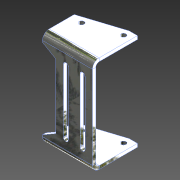
# Autodesk Inventor part: trackball_l
Saved by Autodesk Inventor 2018 (Build 220112000, 112)
## iProperties
Created: 2018-07-04
Part Number: trackball_l
Material: アルミニウム 6061
Document SubType Name: Sheet Metal
Designer: NaMACHAN
Mass: 10.2075 g
Surface Area: 46.6968 cm^2
Volume: 3.78056 cm^3
Density: 2.7 g/cm^3
Sheet Metal Rule: Default
Appearance: アルミニウム - フラット
Author: NaMACHAN
Autodesk Inventor part; units mm, degrees
ref_plane "YZ Plane" through (0, 0, 0) normal (1, 0, 0) x (0, 1, 0)
ref_plane "XZ Plane" through (0, 0, 0) normal (0, 1, 0) x (-1, 0, 0)
ref_plane "XY Plane" through (0, 0, 0) normal (0, 0, 1) x (1, 0, 0)
sketch "スケッチ1" plane through (0, 0, 0) normal (0, 1, 0) x (-1, 0, 0)
  line L0 (-15, -27) -> (15, -27)
  line L1 (15, 27) -> (-15, 27)
  line L2 (-15, 27) -> (-15, -27)
  line L3 (-15, -27) -> (15, 27) construction
  line L4 (15, -27) -> (-15, 27) construction
  line L5 (15, -27) -> (15, -24)
  line L6 (15, -24) -> (7, -19.3812)
  line L7 (7, -19.3812) -> (7, 19.3812)
  line L8 (7, 19.3812) -> (15, 24)
  line L9 (15, 24) -> (15, 27)
  point P0 (0, 0)
  dimension "d0" = 30
  dimension "d1" = 54
  dimension "d36" = 120
  dimension "d37" = 120
  dimension "d38" = 3
  dimension "d39" = 8
  dimension "d43" = 3
  measures "d0" distance of L1.end L1.start
  measures "d1" distance of L1.start L0.end
  measures "d36" angle of L5 L6
  measures "d37" angle of L9 L8
  measures "d38" distance of L1.start L8.end
  measures "d39" distance between parallel lines of L9 L7
  measures "d43" distance of L0.end L5.end
extrude "プレート1" add sketch "スケッチ1" along normal blind 2
sketch "スケッチ2" plane through (-15, 0, 27) normal (0, 0, 1) x (1, 0, 0)
  line L0 (0, 2) -> (30, 2)
  line L1 (0, 2) -> (0, 12)
  line L2 (0, 12) -> (25, 23)
  line L3 (25, 23) -> (30, 23)
  line L4 (30, 23) -> (30, 2)
  line L5 (0, 0) -> (0, 2)
  line L6 (30, 2) -> (0, 2)
  point P0 (15, 0)
  dimension "d3" = 10
  dimension "d4" = 5
  dimension "d5" = 21
  measures "d3" distance of L0.start L1.end
  measures "d4" distance of L2.end L3.end
  measures "d5" distance between parallel lines of L3 L0
sheet face with bend "面2" sketch "スケッチ2" thickness 2 toward (0, 0, 1) bend radius 2 relief tear relief width 2 relief depth 1
bend "曲げ1"
sketch "スケッチ3" plane through (15, 0, -27) normal (0, 0, -1) x (-1, 0, 0)
  line L0 (0, 0) -> (0, 2)
  line L1 (0, 2) -> (0, 23)
  line L2 (0, 23) -> (5, 23)
  line L3 (0, 23) -> (5, 23)
  line L4 (30, 12) -> (30, 4)
  line L5 (5, 23) -> (30, 12)
  line L6 (30, 0) -> (30, 2)
  line L7 (30, 12) -> (30, 2)
  line L8 (30, 2) -> (0, 2)
  point P0 (15, 0)
sheet face with bend "面3" sketch "スケッチ3" thickness 2 toward (0, 0, -1) bend radius 2 relief tear relief width 2 relief depth 1
bend "曲げ2"
sketch "スケッチ4" plane through (15, 0, -29) normal (0, 0, -1) x (-1, 0, 0)
  line L0 (5, 23) -> (30, 12) projected
  line L1 (0, 23) -> (5, 23) projected
  point P0 (15, 0)
  point P1 (4.1589, 19)
  point P2 (22.4652, 10.9452)
  dimension "d16" = 4
  dimension "d17" = 4
  dimension "d18" = 20
  dimension "d19" = 4
  measures "d16" distance from line of L0 point (22.465, 10.945)
  measures "d17" distance from line of L0 point (4.159, 19)
  measures "d18" distance of point (4.159, 19) point (22.465, 10.945)
  measures "d19" distance from line of L1 point (4.159, 19)
hole "穴1" at (10.8411, 19, -29) at (-7.4652, 10.9452, -29) direction (0, 0, 1) diameter 3 end through all
sketch "スケッチ5" plane through (0, 2, 0) normal (0, 1, 0) x (1, 0, 0)
  line L0 (10.5, 19) -> (10.5, -19)
  arc A0 (7.5, -19) -> (10.5, -19) centre (9, -19) ccw
  line L1 (7.5, -19) -> (7.5, 19)
  arc A1 (10.5, 19) -> (7.5, 19) centre (9, 19) ccw
  line L2 (0.5, 19) -> (0.5, -19)
  arc A2 (-2.5, -19) -> (0.5, -19) centre (-1, -19) ccw
  line L3 (-2.5, -19) -> (-2.5, 19)
  arc A3 (0.5, 19) -> (-2.5, 19) centre (-1, 19) ccw
  line L4 (15, 25) -> (15, -25) projected
  line L5 (15, 25) -> (-15, 25) projected
  line L6 (-15, -25) -> (15, -25) projected
  line L7 (-15, 24) -> (-15, 25) projected
  point P0 (0, 0)
  point P1 (-15, -26)
  point P2 (-15, 26)
  dimension "d27" = 6
  dimension "d30" = 1.5
  dimension "d31" = 1.5
  dimension "d32" = 6
  dimension "d33" = 6
  dimension "d41" = 14
  constraints: 8 end point, 8 point on circle, 6 tangent, 4 centre point, 4 horizontal alignment, 2 vertical, 1 parallel, 1 vertical alignment, 2 other
  measures "d27" distance from line of L4 A1.centre
  measures "d30" radius of A3
  measures "d31" radius of A1
  measures "d41" distance from line of A3.centre L7
extrude "押し出し1" cut sketch "スケッチ5" against normal blind 10
equation "\"d25\" = Thickness"
equation "\"d2\" = Thickness"
equation "\"d6\" = BendRadius"
equation "\"d7\" = BendReliefWidth"
equation "\"d9\" = MinimumRemnant"
equation "\"d8\" = BendReliefDepth"
equation "\"d10\" = TransitionRadius"
equation "\"d11\" = BendRadius"
equation "\"d12\" = BendReliefWidth"
equation "\"d14\" = MinimumRemnant"
equation "\"d13\" = BendReliefDepth"
equation "\"d15\" = TransitionRadius"
equation "\"BendRadius\" = Thickness"
equation "\"BendReliefWidth\" = Thickness"
equation "\"BendReliefDepth\" = 0.5 * Thickness"
equation "\"CornerReliefSize\" = 4 * Thickness"
equation "\"MinimumRemnant\" = 2 * Thickness"
equation "\"TransitionRadius\" = BendRadius"
equation "\"JacobiRadiusSize\" = Thickness"
equation "\"GapSize\" = Thickness"
equation "\"Thickness\" = 2"
